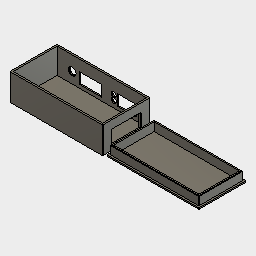
Alt Box v1 (Autodesk Fusion 360 design; units mm, degrees)
Autodesk Fusion 360 part; units mm, degrees
sketch "Sketch1" plane through (0, 0, 0) normal (0, 1, 0) x (1, 0, 0)
  line L0 (10, -10) -> (10, -66)
  line L1 (10, -10) -> (120, -10)
  line L2 (10, -66) -> (120, -66)
  line L3 (120, -66) -> (120, -10)
  dimension "d2" = 56
  measures "d2" distance of L0.start L0.end
extrude "Extrude1" add sketch "Sketch1" along normal blind 2 makes body 1
sketch "Sketch2" plane through (0, 2, 0) normal (0, 1, 0) x (-1, 0, 0)
  line L0 (-10, 10) -> (-10, 66)
  line L1 (-10, 66) -> (-120, 66)
  line L2 (-120, 66) -> (-120, 10)
  line L3 (-120, 10) -> (-10, 10)
  line L4 (-10, 10) -> (-10, 66)
  line L5 (-10, 66) -> (-120, 66)
  line L6 (-120, 66) -> (-120, 10)
  line L7 (-120, 10) -> (-10, 10)
  line L8 (-12, 12) -> (-12, 64)
  line L9 (-12, 64) -> (-118, 64)
  line L10 (-118, 64) -> (-118, 12)
  line L11 (-118, 12) -> (-12, 12)
extrude "Extrude2" add sketch "Sketch2" along normal blind 30 bodies 1
sketch "Sketch3" plane through (120, 0, 0) normal (1, 0, 0) x (0, 0, -1)
  line L0 (-66, 0) -> (-10, 0)
  line L1 (-10, 0) -> (-10, 32)
  line L2 (-10, 32) -> (-66, 32)
  line L3 (-66, 32) -> (-66, 0)
  line L4 (-55, 6) -> (-21, 6)
  line L5 (-55, 22) -> (-21, 22)
  line L6 (-55, 22) -> (-55, 6)
  line L7 (-21, 22) -> (-21, 6)
extrude "Extrude3" cut sketch "Sketch3" against normal blind 5 contours L4 L5 L6 L7 bodies 1
sketch "Sketch4" plane through (0, 0, 10) normal (0, 0, -1) x (-1, 0, 0)
  line L0 (-120, 0) -> (-10, 0)
  line L1 (-10, 0) -> (-10, 32)
  line L2 (-10, 32) -> (-120, 32)
  line L3 (-120, 32) -> (-120, 0)
  line L4 (-106, 6) -> (-106, 19)
  line L5 (-106, 6) -> (-106, 19)
  line L6 (-106, 19) -> (-83, 19)
  line L7 (-83, 19) -> (-83, 6)
  line L8 (-83, 6) -> (-106, 6)
  line L9 (-65, 19) -> (-65, 6)
  line L10 (-65, 19) -> (-38, 19)
  line L11 (-38, 19) -> (-38, 6)
  line L12 (-38, 6) -> (-65, 6)
  dimension "d17" = 13
  dimension "d18" = 23
  dimension "d19" = 18
  dimension "d20" = 27
  measures "d17" distance of L4.start L4.end
  measures "d18" distance of L4.end L6.end
  measures "d19" distance of L6.end L9.start
  measures "d20" distance of L9.start L10.end
extrude "Extrude4" cut sketch "Sketch4" against normal blind 5 contours L4 L5 L6 L7 L8 | L9 L10 L11 L12 bodies 1
sketch "Sketch5" plane through (0, 0, 10) normal (0, 0, -1) x (-1, 0, 0)
  line L0 (-106, 19) -> (-83, 19)
  line L1 (-83, 19) -> (-83, 6)
  line L2 (-83, 6) -> (-106, 6)
  line L3 (-106, 6) -> (-106, 19)
  line L4 (-38, 6) -> (-65, 6)
  line L5 (-65, 6) -> (-65, 19)
  line L6 (-65, 19) -> (-38, 19)
  line L7 (-38, 19) -> (-38, 6)
  line L8 (-120, 0) -> (-10, 0)
  line L9 (-10, 0) -> (-10, 32)
  line L10 (-10, 32) -> (-120, 32)
  line L11 (-120, 32) -> (-120, 0)
  circle A0 centre (-30, 15) radius 4
  dimension "d23" = 8
  measures "d23" diameter of A0
extrude "Extrude5" cut sketch "Sketch5" against normal blind 5 contours A0 bodies 1
fillet "Fillet1" radius 0.5 1 edges at (33.7293, 13.5535, 12) on bodies 1
fillet "Fillet2" radius 0.5 1 edges at (33.7293, 16.4465, 10) on bodies 1
sketch "Sketch6" plane through (0, 0, 10) normal (0, 0, -1) x (-1, 0, 0)
  line L0 (-120, 0) -> (-10, 0)
  line L1 (-10, 0) -> (-10, 32)
  line L2 (-10, 32) -> (-120, 32)
  line L3 (-120, 32) -> (-120, 0)
  line L4 (-38, 6) -> (-65, 6)
  line L5 (-65, 6) -> (-65, 19)
  line L6 (-65, 19) -> (-38, 19)
  line L7 (-38, 19) -> (-38, 6)
  line L8 (-106, 19) -> (-83, 19)
  line L9 (-83, 19) -> (-83, 6)
  line L10 (-83, 6) -> (-106, 6)
  line L11 (-106, 6) -> (-106, 19)
  circle A0 centre (-30, 15) radius 4.5
  circle A1 centre (-79, 16) radius 2.5
  circle A2 centre (-79.0282, 10) radius 2.5
  dimension "d28" = 5
  dimension "d29" = 5
  measures "d28" diameter of A1
  measures "d29" diameter of A2
extrude "Extrude6" cut sketch "Sketch6" against normal blind 5 contours A1 | A2 bodies 1
fillet "Fillet3" radius 0.5 4 edges at (81.359, 9.096, 12) (81.359, 10.904, 10) (81.3308, 15.096, 12) (81.3308, 16.904, 10) on bodies 1
fillet "Fillet4" radius 0.5 2 edges at (120, 16, 66) (120, 16, 10) on bodies 1
fillet "Fillet5" radius 0.5 2 edges at (10, 16, 10) (10, 16, 66) on bodies 1
fillet "Fillet6" radius 0.5 8 edges at (119.8536, 0, 10.1464) (120, 0, 38) (119.8536, 0, 65.8536) (65, 0, 66) (10.1464, 0, 65.8536) (10, 0, 38) (10.1464, 0, 10.1464) (65, 0, 10) on bodies 1
fillet "Fillet7" radius 0.5 4 edges at (38, 19, 11) (65, 6, 11) (65, 19, 11) (38, 6, 11) on bodies 1
fillet "Fillet8" radius 0.5 8 edges at (64.8536, 18.8536, 10) (51.5, 19, 10) (38.1464, 18.8536, 10) (38, 12.5, 10) (38.1464, 6.1464, 10) (51.5, 6, 10) (64.8536, 6.1464, 10) (65, 12.5, 10) on bodies 1
fillet "Fillet9" radius 0.5 4 edges at (119, 6, 21) (119, 6, 55) (119, 22, 55) (119, 22, 21) on bodies 1
fillet "Fillet10" radius 0.5 8 edges at (120, 21.8536, 21.1464) (120, 14, 21) (120, 6.1464, 21.1464) (120, 6, 38) (120, 6.1464, 54.8536) (120, 14, 55) (120, 21.8536, 54.8536) (120, 22, 38) on bodies 1
fillet "Fillet11" radius 0.5 4 edges at (83, 6, 11) (83, 19, 11) (106, 6, 11) (106, 19, 11) on bodies 1
fillet "Fillet12" radius 0.5 8 edges at (83.1464, 18.8536, 10) (83, 12.5, 10) (83.1464, 6.1464, 10) (94.5, 6, 10) (105.8536, 6.1464, 10) (106, 12.5, 10) (105.8536, 18.8536, 10) (94.5, 19, 10) on bodies 1
sketch "Sketch7" plane through (0, 2, 0) normal (0, 1, 0) x (-1, 0, 0)
  line L0 (-12, 12) -> (-12, 64)
  line L1 (-12, 64) -> (-118, 64)
  line L2 (-118, 64) -> (-118, 12)
  line L3 (-118, 12) -> (-12, 12)
  line L4 (-125, 10) -> (-125, 66)
  line L5 (-125, 66) -> (-234, 66)
  line L6 (-125, 10) -> (-234, 10)
  line L7 (-234, 10) -> (-234, 66)
  dimension "d42" = 109
  dimension "d43" = 109
  measures "d42" distance of L4.end L5.end
  measures "d43" distance of L4.start L6.end
extrude "Extrude7" add sketch "Sketch7" along normal blind 2 separate body contours L4 L5 L6 L7 makes body 2
sketch "Sketch8" plane through (0, 4, 0) normal (0, 1, 0) x (-1, 0, 0)
  line L0 (-125, 10) -> (-125, 66)
  line L1 (-125, 66) -> (-234, 66)
  line L2 (-234, 66) -> (-234, 10)
  line L3 (-234, 10) -> (-125, 10)
  line L4 (-127.1, 63.9) -> (-231.9, 63.9)
  line L5 (-231.9, 63.9) -> (-231.9, 12.1)
  line L6 (-231.9, 12.1) -> (-127.1, 12.1)
  line L7 (-127.1, 12.1) -> (-127.1, 63.9)
  line L8 (-229.9, 14.1) -> (-129.1, 14.1)
  line L9 (-129.1, 61.9) -> (-129.1, 14.1)
  line L10 (-229.9, 14.1) -> (-229.9, 61.9)
  line L11 (-229.9, 61.9) -> (-129.1, 61.9)
  point P0 (-118, 12)
  point P1 (-118, 64)
extrude "Extrude8" add sketch "Sketch8" along normal blind 10 contours L4 L5 L6 L7 bodies 2
fillet "Fillet13" radius 0.5 4 edges at (234, 3, 66) (234, 3, 10) (125, 3, 66) (125, 3, 10) on bodies 2
fillet "Fillet14" radius 0.5 4 edges at (127.1, 9, 12.1) (231.9, 9, 12.1) (231.9, 9, 63.9) (127.1, 9, 63.9) on bodies 2
fillet "Fillet15" radius 0.5 8 edges at (233.8536, 2, 65.8536) (179.5, 2, 66) (125.1464, 2, 65.8536) (125, 2, 38) (125.1464, 2, 10.1464) (179.5, 2, 10) (233.8536, 2, 10.1464) (234, 2, 38) on bodies 2
fillet "Fillet16" radius 0.5 8 edges at (231.7536, 14, 63.7536) (231.9, 14, 38) (231.7536, 14, 12.2464) (179.5, 14, 12.1) (127.2464, 14, 12.2464) (127.1, 14, 38) (127.2464, 14, 63.7536) (179.5, 14, 63.9) on bodies 2
